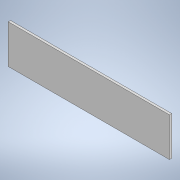
# Autodesk Inventor part: back
Saved by Autodesk Inventor 2021 (Build 250183000, 183)
## iProperties
Created: 2020-07-28
Part Number: back
Material: Generic
Document SubType Name: Modeling
Designer: johna
Density: 1 g/cm^3
Appearance: Default
Author: johna
Autodesk Inventor part; units mm, degrees
ref_plane "YZ Plane" through (0, 0, 0) normal (1, 0, 0) x (0, 1, 0)
ref_plane "XZ Plane" through (0, 0, 0) normal (0, 1, 0) x (-1, 0, 0)
ref_plane "XY Plane" through (0, 0, 0) normal (0, 0, 1) x (1, 0, 0)
sketch "Sketch1" plane through (0, 0, 0) normal (0, 0, 1) x (1, 0, 0)
  line L0 (-26.3498, 6.4797) -> (151.4502, 6.4797)
  line L1 (151.4502, 6.4797) -> (151.4502, -36.2685)
  line L2 (151.4502, -36.2685) -> (-26.3498, -36.2685)
  line L3 (-26.3498, -36.2685) -> (-26.3498, 6.4797)
  point P0 (0, 0)
  dimension "d0" = 177.8
  dimension "d1" = 42.7482
  constraints: 8 end point, 2 parallel, 1 horizontal, 1 perpendicular
  measures "d0" distance of L1.end L2.end
  measures "d1" distance of L0.end L1.end
extrude "Extrusion1" add sketch "Sketch1" along normal blind 2.54
body "Solid1"
